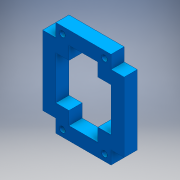
# Autodesk Inventor part: bottomplate
Saved by Autodesk Inventor 2016 (Build 200138000, 138)
## iProperties
Created: 2016-06-11
Part Number: bottomplate
Material: Generic
Document SubType Name: Modeling
Designer: hesaon
Density: 1 g/cm^3
Appearance: Default
Author: hesaon
Autodesk Inventor part; units mm, degrees
ref_plane "YZ Plane" through (0, 0, 0) normal (1, 0, 0) x (0, 1, 0)
ref_plane "XZ Plane" through (0, 0, 0) normal (0, 1, 0) x (-1, 0, 0)
ref_plane "XY Plane" through (0, 0, 0) normal (0, 0, 1) x (1, 0, 0)
sketch "Sketch1" plane through (0, 0, 0) normal (0, 1, 0) x (-1, 0, 0)
  line L0 (0, 0) -> (42, 0)
  line L1 (42, 0) -> (42, -73)
  line L2 (42, -73) -> (0, -73)
  line L3 (0, -73) -> (0, 0)
  dimension "d0" = 42
  dimension "d1" = 73
  constraints: 8 end point, 2 parallel, 1 horizontal, 1 perpendicular
  measures "d0" distance of L1.end L2.end
  measures "d1" distance of L0.end L1.end
extrude "Extrusion1" add sketch "Sketch1" along normal blind 10
hole "Hole1" at (-37, 10, -5) direction (0, -1, 0) diameter 4.4 end through all
hole "Hole2" at (-37, 10, -68) direction (0, -1, 0) diameter 4.4 end through all
hole "Hole3" at (-5, 10, -68) direction (0, -1, 0) diameter 4.4 end through all
hole "Hole4" at (-5, 10, -5) direction (0, -1, 0) diameter 4.4 end through all
sketch "Sketch2" plane through (0, 0, 0) normal (1, 0, 0) x (0, 0, -1)
  line L0 (10, 10) -> (63, 10)
  line L1 (63, 10) -> (63, 0)
  line L2 (63, 0) -> (10, 0)
  line L3 (10, 0) -> (10, 10)
  line L4 (0, 10) -> (73, 10) projected
  line L5 (73, 0) -> (0, 0) projected
  dimension "d40" = 10
  dimension "d41" = 10
  constraints: 8 end point, 2 collinear, 2 parallel, 1 horizontal, 1 perpendicular
  measures "d40" distance of L4.start L0.start
  measures "d41" distance of L4.end L0.end
extrude "Extrusion2" add sketch "Sketch2" along normal blind 10
sketch "Sketch4" plane through (-42, 0, -73) normal (-1, 0, 0) x (0, 0, 1)
  line L0 (10, 10) -> (63, 10)
  line L1 (63, 10) -> (63, 0)
  line L2 (63, 0) -> (10, 0)
  line L3 (10, 0) -> (10, 10)
  line L4 (73, 0) -> (0, 0) projected
  line L5 (0, 10) -> (73, 10) projected
  dimension "d44" = 10
  dimension "d45" = 10
  constraints: 8 end point, 2 collinear, 2 parallel, 1 horizontal, 1 perpendicular
  measures "d44" distance of L5.end L0.end
  measures "d45" distance of L0.start L5.start
extrude "Extrusion3" add sketch "Sketch4" along normal blind 10
sketch "Sketch5" plane through (0, 10, 0) normal (0, 1, 0) x (1, 0, 0)
  line L0 (-42, 53) -> (0, 53)
  line L1 (0, 53) -> (0, 20)
  line L2 (0, 20) -> (-42, 20)
  line L3 (-42, 20) -> (-42, 53)
  line L4 (10, 63) -> (10, 10) projected
  line L5 (0, 73) -> (-42, 73) projected
  line L6 (-52, 10) -> (-52, 63) projected
  point P0 (0, 0)
  dimension "d48" = 10
  dimension "d49" = 20
  dimension "d50" = 20
  dimension "d51" = 10
  constraints: 8 end point, 2 parallel, 1 horizontal, 1 perpendicular
  measures "d48" distance from line of L4 L0.end
  measures "d49" distance of point (0, 0) L1.end
  measures "d50" distance from line of L5 L0.end
  measures "d51" distance from line of L6 L0.start
extrude "Extrusion4" cut sketch "Sketch5" against normal up to next
sketch "Sketch6" plane through (0, 10, 0) normal (0, 1, 0) x (1, 0, 0)
  line L0 (-32, 63) -> (-10, 63)
  line L1 (-10, 63) -> (-10, 53)
  line L2 (-10, 53) -> (-32, 53)
  line L3 (-32, 53) -> (-32, 63)
  line L4 (-32, 20) -> (-10, 20)
  line L5 (-10, 20) -> (-10, 10)
  line L6 (-10, 10) -> (-32, 10)
  line L7 (-32, 10) -> (-32, 20)
  line L8 (-42, 53) -> (0, 53) projected
  line L9 (0, 20) -> (-42, 20) projected
  line L10 (0, 63) -> (0, 73) projected
  line L11 (-42, 73) -> (-42, 63) projected
  line L12 (0, 0) -> (0, 10) projected
  line L13 (-42, 10) -> (-42, 0) projected
  line L14 (-42, 63) -> (-52, 63) projected
  line L15 (0, 10) -> (10, 10) projected
  dimension "d54" = 10
  dimension "d55" = 10
  dimension "d56" = 10
  dimension "d57" = 10
  constraints: 16 end point, 4 collinear, 4 parallel, 2 horizontal, 2 perpendicular
  measures "d54" distance between parallel lines of L10 L1
  measures "d55" distance between parallel lines of L11 L3
  measures "d56" distance between parallel lines of L12 L5
  measures "d57" distance between parallel lines of L13 L7
extrude "Extrusion5" cut sketch "Sketch6" against normal up to next
body "Solid1"
